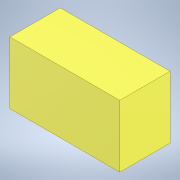
# Autodesk Inventor part: poeAdapter
Saved by Autodesk Inventor 2022.1 (Build 261234000, 234)
## iProperties
Created: 2021-08-20
Part Number: poeAdapter
Material: PC/ABS Plastic
Document SubType Name: Modeling
Designer: robst
Density: 0.357273 g/cm^3
Appearance: Smooth - Yellow
Author: robst
Autodesk Inventor part; units mm, degrees
ref_plane "YZ Plane" through (0, 0, 0) normal (1, 0, 0) x (0, 1, 0)
ref_plane "XZ Plane" through (0, 0, 0) normal (0, 1, 0) x (-1, 0, 0)
ref_plane "XY Plane" through (0, 0, 0) normal (0, 0, 1) x (1, 0, 0)
sketch "Sketch8" plane through (0, 0, 0) normal (0, 0, 1) x (1, 0, 0)
  line L0 (-41.5, -23.5) -> (41.5, -23.5)
  line L1 (41.5, -23.5) -> (41.5, 23.5)
  line L2 (41.5, 23.5) -> (-41.5, 23.5)
  line L3 (-41.5, 23.5) -> (-41.5, -23.5)
  line L4 (-41.5, -23.5) -> (41.5, 23.5) construction
  line L5 (41.5, -23.5) -> (-41.5, 23.5) construction
  point P0 (0, 0)
  dimension "d31" = 47
  dimension "d32" = 83
  constraints: 12 end point, 2 midpoint, 2 parallel, 1 horizontal, 1 perpendicular
  measures "d31" distance of L0.end L1.end
  measures "d32" distance of L1.end L2.end
extrude "Extrusion6" add sketch "Sketch8" against normal blind 38
equation "\"d31\" = poeWidth"
equation "\"d32\" = poeLength"
equation "\"d33\" = poeDepth"
equation "\"wallThickness\" = 5"
equation "\"caseWidth\" = piCaseLength + 2 * wallThickness"
equation "\"oneHalfCaseDepth\" = 0.5 * fanWidth + wallThickness"
equation "\"caseLength\" = 189.7"
equation "\"cameraLength\" = 55"
equation "\"lensLength\" = 15.7"
equation "\"piCaseWidth\" = 65"
equation "\"piCaseDepth\" = 32"
equation "\"poeLength\" = 83"
equation "\"poeWidth\" = 47"
equation "\"poeDepth\" = 38"
equation "\"piEthernetCableReliefLength\" = 35"
equation "\"piCaseLength\" = 129"
equation "\"fanWidth\" = 60"
body "Solid2"
